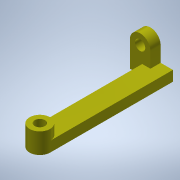
# Autodesk Inventor part: 本體
Saved by Autodesk Inventor 2022 (Build 260153000, 153)
## iProperties
Created: 2020-03-26
Part Number: 本體
Material: 一般
Document SubType Name: Modeling
Designer: Kuan-Lun Hsu
Density: 1 g/cm^3
Appearance: 黃
Author: Kuan-Lun Hsu
Autodesk Inventor part; units mm, degrees
ref_plane "YZ Plane" through (0, 0, 0) normal (1, 0, 0) x (0, 1, 0)
ref_plane "XZ Plane" through (0, 0, 0) normal (0, 1, 0) x (-1, 0, 0)
ref_plane "XY Plane" through (0, 0, 0) normal (0, 0, 1) x (1, 0, 0)
sketch "草圖1" plane through (0, 0, 0) normal (0, 0, 1) x (1, 0, 0)
  line L0 (-10, 120) -> (10, 120)
  line L1 (10, 120) -> (10, -20)
  line L2 (10, -20) -> (-10, -20)
  line L3 (-10, -20) -> (-10, 120)
  line L4 (10, 110) -> (-10, 110)
  line L5 (10, 120) -> (10, 110)
  line L6 (-10, 110) -> (-22, 110)
  line L7 (-22, 110) -> (-22, 120)
  line L8 (-22, 120) -> (-10, 120)
  line L9 (-10, 120) -> (-10, 110)
  line L10 (10, 110) -> (22, 110)
  line L11 (22, 110) -> (22, 120)
  line L12 (22, 120) -> (10, 120)
  line L13 (10, 120) -> (10, 110)
  point P0 (0, 0)
  point P1 (0, -20)
  dimension "d0" = 20
  dimension "d1" = 140
  dimension "d2" = 20
  dimension "d18" = 10
  dimension "d20" = 12
  dimension "d21" = 10
  dimension "d22" = 12
  dimension "d23" = 10
  constraints: 28 end point, 6 parallel, 4 perpendicular, 3 horizontal, 2 point on line, 1 midpoint, 1 vertical alignment
  measures "d0" distance from line of L2 point (0, 0)
  measures "d1" distance of L2.end L0.start
  measures "d2" distance of L0.start L0.end
  measures "d18" distance between parallel lines of L0 L4
  measures "d20" distance between parallel lines of L3 L7
  measures "d21" distance between parallel lines of L6 L8
  measures "d22" distance of L4.start L10.end
  measures "d23" distance between parallel lines of L10 L12
extrude "擠出1" add sketch "草圖1" along normal blind 10 contours L0 L1 L4 L3 | L3 L6 L7 L8 | L4 L1 L2 L3
sketch "草圖2" plane through (0, 0, 10) normal (0, 0, 1) x (1, 0, 0)
  circle A0 centre (0, 0) radius 10
  circle A1 centre (0, 0) radius 5
  dimension "d5" = 20
  dimension "d6" = 10
  constraints: 2 centre point, 2 coincident
  measures "d5" diameter of A0
  measures "d6" diameter of A1
extrude "擠出2" add sketch "草圖2" along normal blind 10
sketch "草圖3" plane through (-10, 120, 0) normal (0, 1, 0) x (1, 0, 0)
  circle A0 centre (-2, -25) radius 10
  line L0 (20, -10) -> (-12, -10) projected
  line L1 (-12, 0) -> (20, 0) projected
  line L2 (-12, 0) -> (8, 0)
  line L3 (8, 0) -> (8, -25)
  line L4 (8, -25) -> (-12, -25)
  line L5 (-12, -25) -> (-12, 0)
  line L6 (-12, 0) -> (-12, -10) projected
  point P0 (10, 0)
  point P1 (0, -10)
  point P2 (0, 0)
  point P3 (32, -10)
  point P4 (32, 0)
  point P5 (8, -10)
  dimension "d9" = 20
  dimension "d10" = 25
  constraints: 8 end point, 2 parallel, 2 point on circle, 1 centre point, 1 collinear, 1 horizontal, 1 perpendicular, 1 tangent
  measures "d9" diameter of A0
  measures "d10" distance from line of L1 A0.centre
extrude "擠出3" add sketch "草圖3" against normal blind 10 contours L4 A0 | A0 L5 L0 L3 | A0 L4
sketch "草圖4" plane through (-10, 120, 0) normal (0, 1, 0) x (1, 0, 0)
  circle A0 centre (-2, -25) radius 10 projected
  circle A1 centre (-2, -25) radius 5
  point P0 (10, 0)
  point P1 (8, -25)
  point P2 (-12, -25)
  point P3 (0, 25)
  dimension "d13" = 10
  constraints: 1 centre point, 1 coincident, 1 other
  measures "d13" diameter of A1
extrude "擠出4" cut sketch "草圖4" against normal blind 10 contours A1
sketch "草圖5" plane through (0, 0, 10) normal (0, 0, 1) x (1, 0, 0)
  arc A0 (-10, 0) -> (10, 0) centre (0, 0) ccw projected
  line L0 (-10, 0) -> (-10, -20) projected
  line L1 (-10, -20) -> (10, -20) projected
  line L2 (10, -20) -> (10, 0) projected
extrude "擠出5" cut sketch "草圖5" against normal through all
equation "\"d21\" = d18"
equation "\"d22\" = d20"
equation "\"d23\" = d21"
